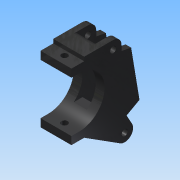
# Autodesk Inventor part: Front Axle Housing
Saved by Autodesk Inventor 2014 (Build 180170000, 170)
## iProperties
Created: 2014-01-04
Part Number: Front Axle Housing
Material: ABS Plastic
Document SubType Name: Modeling
Designer: davidgitz
Density: 1.06 g/cm^3
Appearance: Dark Gray
Author: davidgitz
Autodesk Inventor part; units mm, degrees
ref_plane "YZ Plane" through (0, 0, 0) normal (1, 0, 0) x (0, 1, 0)
ref_plane "XZ Plane" through (0, 0, 0) normal (0, 1, 0) x (-1, 0, 0)
ref_plane "XY Plane" through (0, 0, 0) normal (0, 0, 1) x (1, 0, 0)
sketch "Sketch1" plane through (0, 0, 0) normal (1, 0, 0) x (0, 1, 0)
  arc A0 (39.954, 1.6866) -> (44.513, 5.9979) centre (40.195, 5.9979) ccw
  circle A1 centre (40.195, 5.9979) radius 1.5875
  line L0 (44.513, 5.9979) -> (44.513, 20.9839)
  line L1 (44.513, 20.9839) -> (42.481, 20.9839)
  line L2 (42.481, 20.9839) -> (42.481, 27.5879)
  line L3 (42.481, 27.5879) -> (38.417, 27.5879)
  line L4 (38.417, 27.5879) -> (38.417, 23.5239)
  line L5 (39.954, 1.6866) -> (37.414, 1.6866)
  line L6 (37.414, 1.6866) -> (36.4393, -3.299)
  line L7 (36.4393, -3.299) -> (10.8933, -7.6145)
  line L8 (10.8933, -7.6145) -> (7.2025, -0.948)
  line L9 (7.2025, -0.948) -> (2.0915, -3.7777)
  arc A2 (-3.6468, 2.3121) -> (2.0915, -3.7777) centre (0, 0) ccw
  circle A3 centre (0, 0) radius 1.5875
  line L10 (8.191, 27.5879) -> (12.255, 27.5879)
  line L11 (12.255, 27.5879) -> (12.255, 23.5239)
  arc A4 (12.255, 23.5239) -> (38.417, 23.5239) centre (25.336, 23.5239) ccw
  line L12 (81.5814, 1.6799) -> (58.7298, 1.6799) construction
  line L13 (40.195, 5.9979) -> (0, 0) construction
  line L14 (8.191, 27.5879) -> (10.8933, -7.6145) construction
  line L15 (60.3567, 10.4429) -> (44.3212, 10.4429) construction
  line L16 (8.191, 27.5879) -> (0, 0) construction
  line L17 (-6.8832, 3.5179) -> (4.3798, -16.8256) construction
  line L18 (8.191, 27.5879) -> (8.191, 20.9839)
  line L19 (8.191, 20.9839) -> (-3.6468, 2.3121)
  dimension "d0" = 8.636
  dimension "d1" = 3.175
  dimension "d2" = 4.064
  dimension "d3" = 6.604
  dimension "d4" = 2.032
  dimension "d5" = 25.908
  dimension "d6" = 2.54
  dimension "d7" = 5.08
  dimension "d8" = 25.908
  dimension "d9" = 7.62
  dimension "d10" = 40.64
  dimension "d11" = 35.306
  dimension "d12" = 26.162
  dimension "d13" = 17.145
  dimension "d14" = 28.7782
  dimension "d15" = 10.16
  constraints: 40 end point, 8 tangent, 6 perpendicular, 6 point on circle, 5 centre point, 5 parallel, 3 coincident, 2 equal length, 2 equal radius, 1 collinear, 1 vertical
  measures "d0" diameter of A0
  measures "d1" diameter of A1
  measures "d2" distance of L2.end L3.end
  measures "d3" distance of L1.end L2.end
  measures "d4" distance of L0.end L1.end
  measures "d5" distance between parallel lines of L12 L3
  measures "d6" distance of L5.start L5.end
  measures "d7" distance of L5.end L6.end
  measures "d8" distance of L6.end L7.end
  measures "d9" distance of L7.end L8.end
  measures "d10" distance of L13.start L13.end
  measures "d11" distance of L10.start L7.end
  measures "d12" distance between parallel lines of L11 L4
  measures "d13" distance between parallel lines of L10 L15
  measures "d14" distance of L10.start L13.end
  measures "d15" distance between parallel lines of L17 L8
extrude "Extrusion1" add sketch "Sketch1" along normal mid plane 16.002
sketch "Sketch2" plane through (0, 0, 0) normal (1, 0, 0) x (0, 1, 0)
  line L0 (38.417, 27.5879) -> (42.481, 27.5879) projected
  line L1 (8.191, 27.5879) -> (12.255, 27.5879) projected
  line L2 (41.338, 10.4429) -> (11.366, 10.4429)
  line L3 (44.513, 20.9839) -> (44.513, 5.9979) projected
  arc A0 (41.338, 10.4429) -> (44.513, 13.6179) centre (41.338, 13.6179) ccw
  line L4 (8.191, 27.5879) -> (8.191, 13.6179)
  arc A1 (8.191, 13.6179) -> (11.366, 10.4429) centre (11.366, 13.6179) ccw
  line L5 (44.513, 13.6179) -> (46.9295, 13.6179)
  line L6 (46.9295, 13.6179) -> (49.0826, -15.2272)
  line L7 (49.0826, -15.2272) -> (-26.66, -17.9242)
  line L8 (-26.66, -17.9242) -> (-26.66, 23.5652)
  line L9 (-26.66, 23.5652) -> (8.191, 27.5879)
  point P0 (0, 0)
  point P1 (44.513, 3.2824)
  dimension "d18" = 17.145
  dimension "d19" = 3.175
  dimension "d20" = 3.175
  constraints: 14 end point, 4 point on circle, 3 tangent, 2 centre point, 2 perpendicular, 1 parallel, 1 point on line
  measures "d18" distance between parallel lines of L2 L0
  measures "d19" radius of A0
  measures "d20" radius of A1
extrude "Extrusion2" cut sketch "Sketch2" along normal mid plane 10.16
sketch "Sketch3" plane through (-8.001, 38.417, 27.5879) normal (0, 0, 1) x (1, 0, 0)
  line L0 (16.002, -26.162) -> (0, -26.162) projected
  line L1 (16.002, -30.226) -> (0, -30.226) projected
  line L2 (0, -30.226) -> (0, -26.162) projected
  line L3 (16.002, -26.162) -> (16.002, -30.226) projected
  line L4 (0, 4.064) -> (16.002, -30.226) construction
  line L5 (4.572, -3.175) -> (11.43, -3.175)
  line L6 (11.43, -3.175) -> (11.43, -22.987)
  line L7 (11.43, -22.987) -> (4.572, -22.987)
  line L8 (4.572, -22.987) -> (4.572, -3.175)
  line L9 (11.43, -3.175) -> (4.572, -22.987) construction
  point P0 (8.001, -38.417)
  point P1 (8.001, -13.081)
  dimension "d23" = 6.858
  dimension "d24" = 19.812
  constraints: 12 end point, 2 midpoint, 2 parallel, 1 horizontal, 1 perpendicular
  measures "d23" distance of L5.start L5.end
  measures "d24" distance of L5.end L6.end
extrude "Extrusion3" cut sketch "Sketch3" against normal through all contours L5 L6 L7 L8
sketch "Sketch4" plane through (-8.001, 42.481, 27.5879) normal (0, 1, 0) x (1, 0, 0)
  line L0 (16.002, 0) -> (0, 0) projected
  circle A0 centre (8.362, 4.064) radius 1.5875
  point P0 (8.001, 27.5879)
  dimension "d27" = 3.175
  dimension "d28" = 4.064
  constraints: 1 centre point
  measures "d27" diameter of A0
  measures "d28" distance from line of L0 A0.centre
extrude "Extrusion4" cut sketch "Sketch4" against normal through all
body "Solid1"
